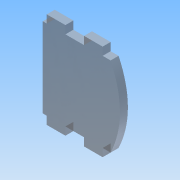
# Autodesk Inventor part: tip
Saved by Autodesk Inventor 2015 (Build 190159000, 159)
## iProperties
Created: 2016-01-28
Part Number: tip
Material: Plastique PMMA
Document SubType Name: Tôlerie
Designer: Gregwar
Density: 1.188 g/cm^3
Sheet Metal Rule: Par défaut_mm
Appearance: Polycarbonate - Transparent
Author: Gregwar
Autodesk Inventor part; units mm, degrees
ref_plane "YZ Plane" through (0, 0, 0) normal (1, 0, 0) x (0, 1, 0)
ref_plane "XZ Plane" through (0, 0, 0) normal (0, 1, 0) x (-1, 0, 0)
ref_plane "XY Plane" through (0, 0, 0) normal (0, 0, 1) x (1, 0, 0)
sketch "Esquisse1" plane through (0, 0, 0) normal (0, 1, 0) x (-1, 0, 0)
  line L0 (0, 0) -> (25.5, 0)
  line L1 (25.5, 0) -> (25.5, -30)
  line L2 (25.5, -30) -> (0, -30)
  line L3 (0, -30) -> (0, 0)
  line L4 (3, 0) -> (10, 0)
  line L5 (10, 0) -> (10, 3)
  line L6 (10, 3) -> (3, 3)
  line L7 (3, 3) -> (3, 0)
  line L8 (25.5, -15) -> (0, -15) construction
  line L9 (14, 0) -> (39.5, 0)
  line L10 (17, 0) -> (24, 0)
  line L11 (24, 0) -> (24, 3)
  line L12 (24, 3) -> (17, 3)
  line L13 (17, 3) -> (17, 0)
  line L14 (3, -30) -> (10, -30)
  line L15 (10, -30) -> (10, -33)
  line L16 (10, -33) -> (3, -33)
  line L17 (3, -33) -> (3, -30)
  line L18 (17, -30) -> (24, -30)
  line L19 (24, -30) -> (24, -33)
  line L20 (24, -33) -> (17, -33)
  line L21 (17, -33) -> (17, -30)
  line L22 (0, 0) -> (-7, -15) construction
  line L23 (-7, -15) -> (0, -30) construction
  spline S0 degree 2 poles (0, 0) (-7, -15) (0, -30) knots 1 1 1 2 2 2
  line L24 (-7, -15) -> (0, -15) construction
  point P0 (14, -30)
  dimension "d0" = 30
  dimension "d1" = 3
  dimension "d2" = 7
  dimension "d3" = 3
  dimension "d6" = 14
  dimension "d11" = 1.5
  dimension "d12" = 7
  measures "d0" distance of L0.end L1.end
  measures "d1" distance between parallel lines of L3 L7
  measures "d2" distance of L5.end L6.end
  measures "d3" distance of L4.end L5.end
  measures "d6" distance of L0.start L9.start
  measures "d11" distance between parallel lines of L11 L1
  measures "d12" distance from line of L22.end L3
extrude "Plaque1" add sketch "Esquisse1" along normal blind 3
equation "\"d6\" = 2 * d2"
equation "\"LargeurGrugeage\" = Epaisseur"
equation "\"ProfondeurGrugeage\" = 0.5 * Epaisseur"
equation "\"TailleGrugeage\" = 4 * Epaisseur"
equation "\"RestesMinimum\" = 2 * Epaisseur"
equation "\"Rayondetransition\" = RayonPli"
equation "\"TailleRayonJacobi\" = RayonPli"
equation "\"TailleJeu\" = Epaisseur"
equation "\"d13\" = RayonPli"
equation "\"Epaisseur\" = 3"
equation "\"RayonPli\" = 4"
